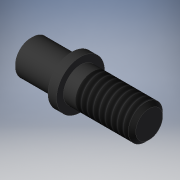
# Autodesk Inventor part: E-NTBGT13-8_b
Saved by Autodesk Inventor 2019 (Build 230136000, 136)
## iProperties
Created: 2024-10-07
Part Number: E-NTBGT13-8_b
Material: Generic
Catalog Web Link: www.cadenas.de
Description: E-NTBG, E-NTSBG, E-NTBGT, E-NTSBGT_base-Economy Bearings with Male Threads
Vendor: MISUMI
Document SubType Name: Modeling
Designer: psAdmin
Manufacturer: MISUMI
Mass: 0.17847 g
Surface Area: 2.32594 cm^2
Volume: 0.17847 cm^3
Density: 1 g/cm^3
Appearance: PSOLRGB-175-175-175
Category: PARTsolutions
Company: MISUMI
Title: E-NTBGT13-8
Author: Cadenas PARTsolutions
Comments: Economy Bearings with Male Threads
PSOL_IDENT_0: {$CADENAS_DATA/23d-libs/misumi/metric/53_rollers/e_ntsbg/e_ntsbg_base.prj},204 {VTYP=3D},{NB=E-NTBGT
PSOL_IDENT_1: 13-8_b},{LINA=E-NTBGT13-8},{NN=E-NTBG, E-NTSBG, E-NTBGT, E-NTSBGT_base},{DATE=17.05.2024 10:16:58},{
PSOL_IDENT_2: GEOMDATE=17.05.2024 10:16:50},{VERSION=},{LINEID=30},{WBVAR=TS,MATB},{WBNUMERIC=}  {NB=E-NTBGT13-8_b
PSOL_IDENT_3: },{LINA=E-NTBGT13-8},{KT=DUMMY},{PN=E-NTBGT13-8},{TYPE=E-NTBGT},{TS=T},{TSALG= '','Standard Male Thr
PSOL_IDENT_4: ead','T','Long Male Thread' },{MATB=},{MATBALG= '','Steel','S','Stainless Steel' },{MATS=Stainless S
PSOL_IDENT_5: teel},{ST=Electroless Nickel Plating},{D=13},{L=8},{B=5.0},{DD=4},{AA=1.0},{G=2.0},{M=M4},{M1=4},{BE=
PSOL_IDENT_6: 624ZZ},{LSM=5},{LLM=8},{D1=5.6},{B1=4.8000},{G1=1.5},{DIA=0.400},{PITCH=0.7},{Z=0.2}
NB: E-NTBGT13-8_b
NN: E-NTBG, E-NTSBG, E-NTBGT, E-NTSBGT_base
NT: Economy Bearings with Male Threads
NBSYN: $PN._b
LINA: E-NTBGT13-8
CATALOG: Misumi
PN: E-NTBGT13-8
TS: Long Male Thread
MATB: Steel
D: 13
L: 8
B: 5
DD: 4
M: M4
SUPPLIER: MISUMI
ARTICLENO: E-NTBGT13-8_b
BOMINFO: E-NTBGT13-8
CREATOR: CADENAS GmbH
Autodesk Inventor part; units mm, degrees
sketch "Sketch_1" plane through (0, 0, 0) normal (0, 0, 1) x (1, 0, 0)
  line L0 (1, 0) -> (-4.8, 0)
  line L1 (-4.8, 0) -> (-4.8, 1.8)
  line L2 (-4.8, 1.8) -> (-4.6, 2)
  line L3 (-4.6, 2) -> (-0.2, 2)
  arc A0 (-0.2, 2) -> (0, 2.2) centre (-0.2, 2.2) ccw
  line L4 (0, 2.2) -> (0, 2.8)
  line L5 (0, 2.8) -> (1, 2.8)
  line L6 (1, 2.8) -> (1, 0)
  line L7 (1, 0) -> (-4.8, 0)
  constraints: 16 end point, 2 point on circle, 1 centre point
revolve "Revolution1" add sketch "Sketch_1" angle 360 about axis through (1, 0, 0) along (1, 0, 0)
sketch "Sketch_5" plane through (0, 0, 0) normal (0, 0, 1) x (1, 0, 0)
  line L0 (9, 0) -> (1, 0)
  line L1 (1, 0) -> (1, 2)
  line L2 (1, 2) -> (8.5705, 2)
  line L3 (8.5705, 2) -> (9, 1.5705)
  line L4 (9, 1.5705) -> (9, 0)
  line L5 (9, 0) -> (1, 0)
  constraints: 12 end point
revolve "Revolution2" add sketch "Sketch_5" angle 360 about axis through (9, 0, 0) along (1, 0, 0)
thread "Thread1" size "M4x0.7" class "6g" standard "ISO Metric profile" length 6.1705
sketch "Sketch_2" plane through (-4.8, 0, 0) normal (1, 0, 0) x (0, 0, -1)
  line L0 (-1, -0.5774) -> (0, -1.1547)
  line L1 (0, -1.1547) -> (1, -0.5774)
  line L2 (1, -0.5774) -> (1, 0.5774)
  line L3 (1, 0.5774) -> (0, 1.1547)
  line L4 (0, 1.1547) -> (-1, 0.5774)
  line L5 (-1, 0.5774) -> (-1, -0.5774)
  constraints: 12 end point
extrude "Extrusion1" cut sketch "Sketch_2" along normal blind 1.5
sketch "Sketch_3" plane through (0, 0, 0) normal (0, 0, 1) x (1, 0, 0)
  line L0 (-2.7226, 0) -> (-3.3, 0)
  line L1 (-3.3, 0) -> (-3.3, 1)
  line L2 (-3.3, 1) -> (-2.7226, 0)
  line L3 (-2.7226, 0) -> (-3.3, 0)
  constraints: 8 end point
revolve "Revolution3" cut sketch "Sketch_3" angle 360 about axis through (-2.7226, 0, 0) along (1, 0, 0)
ref_plane "shaft_to_bearing_XY" through (0, 0, 0) normal (1, 0, 0) x (0, 0, -1)
ref_plane "shaft_to_bearing_YZ" through (0, 0, 0) normal (0, 0, -1) x (0, 1, 0)
ref_plane "shaft_to_bearing_ZX" through (0, 0, 0) normal (0, 1, 0) x (1, 0, 0)
body "Solid1"
